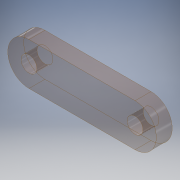
# Autodesk Inventor part: Light gate compression plate
Saved by Autodesk Inventor 2017 (Build 210142000, 142)
## iProperties
Created: 2017-05-18
Part Number: Light gate compression plate
Material: Polycarbonate, Smoke
Document SubType Name: Modeling
Designer: yella
Density: 1.2 g/cm^3
Appearance: Polycarbonate - Smoked
Author: yella
Autodesk Inventor part; units mm, degrees
ref_plane "YZ Plane" through (0, 0, 0) normal (1, 0, 0) x (0, 1, 0)
ref_plane "XZ Plane" through (0, 0, 0) normal (0, 1, 0) x (-1, 0, 0)
ref_plane "XY Plane" through (0, 0, 0) normal (0, 0, 1) x (1, 0, 0)
sketch "Sketch1" plane through (0, 0, 0) normal (0, 1, 0) x (-1, 0, 0)
  circle A0 centre (28, 0) radius 1.5
  circle A1 centre (8, 0) radius 1.5
  arc A2 (28, -4) -> (28, 4) centre (28, 0) ccw
  arc A3 (8, 4) -> (8, -4) centre (8, 0) ccw
  line L0 (28, 4) -> (8, 4)
  line L1 (8, -4) -> (28, -4)
  point P0 (0, 0)
  dimension "d0" = 3
  dimension "d1" = 4
  dimension "d2" = 4
  constraints: 4 centre point, 4 end point, 4 point on circle, 2 coincident, 1 horizontal, 1 parallel, 1 tangent
  measures "d0" diameter of A1
  measures "d1" radius of A2
  measures "d2" radius of A3
extrude "Extrusion1" add sketch "Sketch1" along normal blind 3
body "Solid1"
